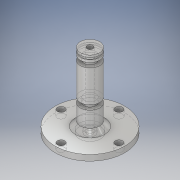
# Autodesk Inventor part: Picker Spool
Saved by Autodesk Inventor 2019.4 (Build 234330000, 330)
## iProperties
Created: 2021-01-08
Part Number: Picker Spool
Material: Generic
Document SubType Name: Modeling
Designer: caleb
Density: 1 g/cm^3
Appearance: Default
Author: caleb
Autodesk Inventor part; units mm, degrees
ref_plane "YZ Plane" through (0, 0, 0) normal (1, 0, 0) x (0, 1, 0)
ref_plane "XZ Plane" through (0, 0, 0) normal (0, 1, 0) x (-1, 0, 0)
ref_plane "XY Plane" through (0, 0, 0) normal (0, 0, 1) x (1, 0, 0)
sketch "Sketch1" plane through (0, 0, 0) normal (0, 1, 0) x (-1, 0, 0)
  circle A0 centre (0, 0) radius 14.2748
  dimension "d0" = 28.5496
  constraints: 1 centre point, 1 coincident
  measures "d0" diameter of A0
extrude "Extrusion1" add sketch "Sketch1" along normal blind 2.3876
sketch "Sketch2" plane through (0, 0, 0) normal (0, -1, 0) x (1, 0, 0)
  circle A0 centre (0, 0) radius 4.3561
  circle A1 centre (0, 0) radius 2.0574
  dimension "d3" = 8.7122
  dimension "d4" = 4.1148
  constraints: 2 centre point, 2 coincident
  measures "d3" diameter of A0
  measures "d4" diameter of A1
extrude "Extrusion2" cut sketch "Sketch2" against normal blind 1.3208
sketch "Sketch3" plane through (0, 2.3876, 0) normal (0, 1, 0) x (1, 0, 0)
  circle A0 centre (0, 0) radius 3.9688
  dimension "d7" = 7.9375
  constraints: 1 centre point, 1 coincident
  measures "d7" diameter of A0
extrude "Extrusion3" add sketch "Sketch3" along normal blind 28.1178
sketch "Sketch4" plane through (0, 30.5054, 0) normal (0, 1, 0) x (1, 0, 0)
  circle A0 centre (0, 0) radius 1.1938
  dimension "d10" = 2.3876
  constraints: 1 centre point, 1 coincident
  measures "d10" diameter of A0
extrude "Extrusion4" cut sketch "Sketch4" against normal through all
chamfer "Chamfer1" distance 2.032 angle 45 1 edges at (-3.9688, 2.3876, 0)
sketch "Sketch5" plane through (0, 0, 0) normal (1, 0, 0) x (0, 1, 0)
  line L0 (4.4196, 3.9688) -> (30.5054, 3.9688) projected
  line L1 (30.5054, -3.9688) -> (30.5054, 3.9688) projected
  line L2 (27.813, 3.9688) -> (25.908, 3.9687)
  line L3 (25.908, 3.9687) -> (25.908, 2.413)
  line L4 (25.908, 2.413) -> (27.813, 2.413)
  line L5 (27.813, 2.413) -> (27.813, 3.9688)
  line L6 (29.5402, 3.9688) -> (28.8036, 3.9688)
  line L7 (28.8036, 3.9688) -> (28.8036, 3.683)
  line L8 (28.8036, 3.683) -> (29.5402, 3.683)
  line L9 (29.5402, 3.683) -> (29.5402, 3.9688)
  line L10 (12.7508, 3.9688) -> (10.8458, 3.9687)
  line L11 (10.8458, 3.9687) -> (10.8458, 2.413)
  line L12 (10.8458, 2.413) -> (12.7508, 2.413)
  line L13 (12.7508, 2.413) -> (12.7508, 3.9688)
  line L14 (-6.1011, 0) -> (36.6065, 0) projected
  point P0 (0, 0)
  dimension "d16" = 0.9652
  dimension "d17" = 0.7366
  dimension "d18" = 0.2858
  dimension "d19" = 2.6924
  dimension "d20" = 1.905
  dimension "d21" = 1.5557
  dimension "d22" = 17.7546
  dimension "d23" = 1.905
  constraints: 24 end point, 6 parallel, 4 point on line, 3 horizontal, 3 perpendicular
  measures "d16" distance between parallel lines of L1 L9
  measures "d17" distance of L7.end L8.end
  measures "d18" distance of L8.end L6.start
  measures "d19" distance between parallel lines of L1 L5
  measures "d20" distance of L3.end L4.end
  measures "d21" distance of L4.end L2.start
  measures "d22" distance between parallel lines of L1 L13
  measures "d23" distance between parallel lines of L11 L13
revolve "Revolution1" cut sketch "Sketch5" angle 360 about axis through (0, -10, 0) along (0, 1, 0)
sketch "Sketch6" plane through (0, 2.3876, 0) normal (0, 1, 0) x (1, 0, 0)
  circle A0 centre (0, 0) radius 1.1938 projected
  circle A1 centre (0, 0) radius 11.8999
  circle A2 centre (-11.8999, 0) radius 1.4986
  circle A3 centre (0, -11.8999) radius 1.4986
  circle A4 centre (11.8999, 0) radius 1.4986
  circle A5 centre (0, 11.8999) radius 1.4986
  dimension "d25" = 23.7998
  dimension "d26" = 2.9972
  dimension "d29" = 360
  constraints: 4 centre point, 1 coincident, 1 horizontal alignment, 11 other
  measures "d26" diameter of A2
extrude "Extrusion5" cut sketch "Sketch6" against normal through all contours A1 A4 | A1 A4 | A5 A1 | A1 A5 | A3 A1 | A1 A3 | A2 A1 | A1 A2
body "Solid1"
